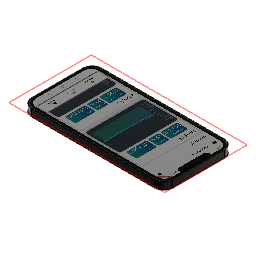
RaumklimaApp v1 (Autodesk Fusion 360 design; units mm, degrees)
Autodesk Fusion 360 part; units mm, degrees
sketch "Skizze1" plane through (0, 0, 0) normal (0, 0, 1) x (1, 0, 0)
  line L0 (0, 0) -> (158, 0)
  line L1 (158, 0) -> (158, 77.8)
  line L2 (158, 77.8) -> (0, 77.8)
  line L3 (0, 77.8) -> (0, 0)
  dimension "d1" = 158
  dimension "d2" = 77.8
  constraint horizontal L0
  constraint vertical L1
  constraint horizontal L2
  constraint vertical L3
  constraint coincident L0.start L3.end
  measures "d1" distance of L0.start L0.end
  measures "d2" distance of L0.start L2.end
extrude "Extrusion1" add sketch "Skizze1" along normal blind 8.1
fillet "Abrundung1" radius 10 4 edges at (0, 0, 4.05) (158, 0, 4.05) (158, 77.8, 4.05) (0, 77.8, 4.05)
